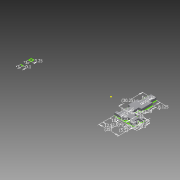
# Autodesk Inventor part: arm-servo
Saved by Autodesk Inventor 2013 (Build 170138000, 138)
## iProperties
Created: 2012-09-08
Part Number: arm-servo
Material: Generic
Document SubType Name: Modeling
Designer: frankenteddy
Density: 1 g/cm^3
Author: frankenteddy
Autodesk Inventor part; units mm, degrees
ref_plane "YZ Plane" through (0, 0, 0) normal (1, 0, 0) x (0, 1, 0)
ref_plane "XZ Plane" through (0, 0, 0) normal (0, 1, 0) x (-1, 0, 0)
ref_plane "XY Plane" through (0, 0, 0) normal (0, 0, 1) x (1, 0, 0)
sketch "Block1" plane through (0, 0, 0) normal (0, 0, 1) x (1, 0, 0)
  circle A0 centre (74.029, 24.2723) radius 1
  line L0 (49.279, 30.4723) -> (71.779, 30.4723)
  line L1 (71.779, 30.4723) -> (71.779, 18.0723)
  line L2 (71.779, 18.0723) -> (49.279, 18.0723)
  line L3 (49.279, 18.0723) -> (49.279, 30.4723)
  line L4 (49.279, 30.4723) -> (44.779, 30.4723)
  line L5 (44.779, 30.4723) -> (44.779, 18.0723)
  line L6 (44.779, 18.0723) -> (49.279, 18.0723)
  line L7 (49.279, 18.0723) -> (49.279, 30.4723)
  line L8 (71.779, 30.4723) -> (76.279, 30.4723)
  line L9 (76.279, 30.4723) -> (76.279, 18.0723)
  line L10 (76.279, 18.0723) -> (71.779, 18.0723)
  line L11 (71.779, 18.0723) -> (71.779, 30.4723)
  line L12 (44.779, 24.2723) -> (76.279, 24.2723) construction
  line L13 (47.029, 30.4723) -> (47.029, 18.0723) construction
  circle A1 centre (47.029, 24.2723) radius 1
  line L14 (74.029, 30.4723) -> (74.029, 18.0723) construction
  point P0 (60.979, 24.0984)
  dimension "d7" = 22.5
  dimension "d8" = 12.4
  dimension "d9" = 4.5
  dimension "d10" = 4.5
  dimension "d11" = 2
  dimension "d12" = 2
  measures "d7" distance of L1.end L2.end
  measures "d8" distance of L0.end L1.end
  measures "d9" distance of L6.end L5.end
  measures "d10" distance of L9.end L10.end
  measures "d11" diameter of A0
  measures "d12" diameter of A1
sketch "Sketch1" plane through (0, 0, 0) normal (0, 0, 1) x (1, 0, 0)
  line L0 (-92.7646, -8.503) -> (-89.7646, -8.503)
  line L1 (-89.7646, -8.503) -> (-89.7646, -11.753)
  line L2 (-89.7646, -11.753) -> (-92.7646, -11.753)
  line L3 (-92.7646, -11.753) -> (-92.7646, -8.503)
  line L4 (-92.7646, -21.6527) -> (-89.7646, -21.6527)
  line L5 (-89.7646, -21.6527) -> (-89.7646, -21.7527)
  line L6 (-89.7646, -21.7527) -> (-92.7646, -21.7527)
  line L7 (-92.7646, -21.7527) -> (-92.7646, -21.6527)
  line L8 (22.861, 24.9107) -> (32.861, 24.9107)
  line L9 (32.861, 24.9107) -> (32.861, -18.3393)
  line L10 (32.861, -18.3393) -> (22.861, -18.3393)
  line L11 (22.861, -18.3393) -> (22.861, 24.9107)
  line L12 (22.861, 24.9107) -> (26.111, 24.9107)
  line L13 (26.111, 24.9107) -> (26.111, 10.9107)
  line L14 (26.111, 10.9107) -> (22.861, 10.9107)
  line L15 (22.861, 10.9107) -> (22.861, 24.9107)
  line L16 (22.861, 3.2857) -> (32.861, 3.2857) construction
  line L17 (26.111, -15.0893) -> (22.861, -15.0893)
  line L18 (26.111, -1.0893) -> (26.111, -15.0893)
  line L19 (22.861, -15.0893) -> (22.861, -1.0893)
  line L20 (22.861, -1.0893) -> (26.111, -1.0893)
  line L21 (32.861, -18.3393) -> (47.861, -18.3393)
  line L22 (47.861, -18.3393) -> (47.861, -5.3393)
  line L23 (47.861, -5.3393) -> (32.861, -5.3393)
  line L24 (32.861, -5.3393) -> (32.861, -18.3393)
  line L25 (47.861, -11.8393) -> (32.861, -11.8393) construction
  line L26 (47.861, -9.3393) -> (44.611, -9.3393)
  line L27 (44.611, -9.3393) -> (44.611, -14.3393)
  line L28 (44.611, -14.3393) -> (47.861, -14.3393)
  line L29 (47.861, -14.3393) -> (47.861, -9.3393)
  line L30 (47.861, -11.8393) -> (44.611, -11.8393) construction
  line L31 (37.861, -5.3393) -> (42.861, -5.3393)
  line L32 (42.861, -5.3393) -> (42.861, -8.5893)
  line L33 (42.861, -8.5893) -> (37.861, -8.5893)
  line L34 (37.861, -8.5893) -> (37.861, -5.3393)
  line L35 (40.361, -5.3393) -> (40.361, -18.3393) construction
  line L36 (40.361, -5.3393) -> (40.361, -8.5893) construction
  line L37 (35.361, -15.0893) -> (42.361, -15.0893)
  line L38 (42.361, -15.0893) -> (42.361, -18.3393)
  line L39 (42.361, -18.3393) -> (35.361, -18.3393)
  line L40 (35.361, -18.3393) -> (35.361, -15.0893)
  line L41 (32.861, 16.7857) -> (36.111, 16.7857)
  line L42 (36.111, 16.7857) -> (36.111, 2.7857)
  line L43 (36.111, 2.7857) -> (32.861, 2.7857)
  line L44 (32.861, 2.7857) -> (32.861, 16.7857)
  point P0 (0, 0)
  dimension "d0" = 3
  dimension "mat" = 3.25
  dimension "d2" = 3
  dimension "d3" = 0.1
  dimension "d32" = 10
  dimension "d33" = 43.25
  dimension "d34" = 3.25
  dimension "d35" = 14
  dimension "d37" = 3.25
  dimension "d38" = 14
  dimension "d40" = 3.25
  dimension "d41" = 15
  dimension "d42" = 13
  dimension "d43" = 3.25
  dimension "d44" = 5
  dimension "d45" = 5
  dimension "d46" = 3.25
  dimension "d47" = 7
  dimension "d48" = 3.25
  dimension "d49" = 12.5
  dimension "d52" = 3.25
  dimension "d53" = 14
  dimension "d54" = 30.25
  dimension "d55" = 8.125
  dimension "d58" = 2.5
  dimension "d59" = 25
  dimension "d60" = 5.5
  constraints: 90 end point, 20 parallel, 10 horizontal, 10 midpoint, 10 perpendicular, 9 collinear
  measures "d0" distance of L1.end L3.start
  measures "mat" distance of L1.start L1.end
  measures "d2" distance of L5.end L7.start
  measures "d3" distance of L5.start L5.end
  measures "d32" distance of L9.end L10.end
  measures "d33" distance of L8.end L9.end
  measures "d34" distance of L14.start L14.end
  measures "d35" distance of L13.start L14.start
  measures "d37" distance of L17.start L17.end
  measures "d38" distance of L18.start L17.start
  measures "d40" distance between parallel lines of L17 L10
  measures "d41" distance of L23.end L22.end
  measures "d42" distance of L22.end L21.end
  measures "d43" distance of L28.end L27.end
  measures "d44" distance of L27.end L26.end
  measures "d45" distance of L32.end L33.end
  measures "d46" distance of L31.end L32.end
  measures "d47" distance of L38.end L39.end
  measures "d48" distance of L37.end L38.end
  measures "d49" distance between parallel lines of L11 L40
  measures "d52" distance of L42.end L43.end
  measures "d53" distance of L41.end L42.end
  measures "d54" distance between parallel lines of L23 L8
  measures "d55" distance between parallel lines of L41 L8
  measures "d58" distance between parallel lines of L40 L24
  measures "d59" distance between parallel lines of L22 L11
  measures "d60" distance between parallel lines of L38 L22
extrude "Extrusion3" add sketch "Sketch1" along normal blind 3.25 contours L8 L9 L10 L11 L17 L18 L20 L14 L13 | L23 L34 L33 L32 L22 L26 L27 L28 L21 L38 L37 L40 L9
extrude "Extrusion4" add sketch "Sketch1" along normal blind 3.25 contours L41 L42 L43 L9
equation "\"d34\" = d36"
equation "\"d37\" = d39"
equation "\"d40\" = mat"
equation "\"d43\" = mat"
equation "\"d46\" = mat"
equation "\"d48\" = mat"
equation "\"d52\" = mat"
equation "\"d50\" = mat"
equation "\"d56\" = mat"
equation "\"d36\" = 3.25"
equation "\"d39\" = 3.25"
body "Solid3"
